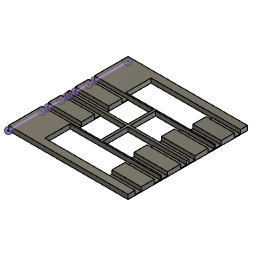
TGI_Display_Peltier_Bracket_ (Autodesk Fusion 360 design; units mm, degrees)
Autodesk Fusion 360 part; units mm, degrees
sketch "スケッチ1" plane through (0, 0, 0) normal (0, 1, 0) x (1, 0, 0)
  line L0 (-50, 50) -> (50, 50)
  line L1 (50, 50) -> (50, -50)
  line L2 (50, -50) -> (-50, -50)
  line L3 (-50, -50) -> (-50, 50)
  constraint horizontal L0
  constraint vertical L1
  constraint horizontal L2
  constraint vertical L3
extrude "押し出し1" add sketch "スケッチ1" along normal blind 3.7
sketch "スケッチ2" plane through (0, 3.7, 0) normal (0, 1, 0) x (-1, 0, 0)
  line L0 (50, 50) -> (-50, 50)
  line L1 (-50, 50) -> (-50, -50)
  line L2 (-50, -50) -> (50, -50)
  line L3 (50, -50) -> (50, 50)
  line L4 (24.7329, -44) -> (-26.2671, -44)
  line L5 (-26.2671, -44) -> (-26.2671, -23)
  line L6 (-26.2671, -23) -> (24.7329, -23)
  line L7 (24.7329, -23) -> (24.7329, -44)
  dimension "d3" = 51
  dimension "d4" = 21
  dimension "d5" = 6
  dimension "d6" = 23.7329
  constraint horizontal L4
  constraint vertical L5
  constraint horizontal L6
  constraint vertical L7
  measures "d3" distance of L4.start L4.end
  measures "d4" distance of L4.start L6.end
  measures "d5" distance of L2 L4
  measures "d6" distance of L1 L5
extrude "押し出し2" cut sketch "スケッチ2" against normal blind 3.7 contours L4 L5 L6 L7
sketch "スケッチ3" plane through (0, 3.7, 0) normal (0, 1, 0) x (-1, 0, 0)
  line L0 (-26.2671, -44) -> (-26.2671, -23)
  line L1 (-26.2671, -23) -> (24.7329, -23)
  line L2 (24.7329, -23) -> (24.7329, -44)
  line L3 (24.7329, -44) -> (-26.2671, -44)
  line L4 (50, 50) -> (-50, 50)
  line L5 (-50, 50) -> (-50, -50)
  line L6 (-50, -50) -> (50, -50)
  line L7 (50, -50) -> (50, 50)
  line L8 (-26.2671, -44) -> (-50.7671, -44)
  line L9 (-50.7671, -44) -> (-50.7671, -39)
  line L10 (-50.7671, -39) -> (-26.2671, -39)
  line L11 (-26.2671, -39) -> (-26.2671, -44)
  line L12 (-26.2671, -23) -> (-50.7671, -23)
  line L13 (-50.7671, -23) -> (-50.7671, -28)
  line L14 (-50.7671, -28) -> (-26.2671, -28)
  line L15 (-26.2671, -28) -> (-26.2671, -23)
  dimension "d9" = 24.5
  dimension "d10" = 5
  dimension "d11" = 24.5
  dimension "d12" = 5
  constraint horizontal L8
  constraint vertical L9
  constraint horizontal L10
  constraint vertical L11
  constraint coincident L0.start L3.end
  constraint horizontal L12
  constraint vertical L13
  constraint horizontal L14
  constraint vertical L15
  constraint coincident L0.end L1.start
  measures "d9" distance of L0.start L8.end
  measures "d10" distance of L0.start L10.end
  measures "d11" distance of L0.end L12.end
  measures "d12" distance of L0.end L14.end
extrude "押し出し3" cut sketch "スケッチ3" against normal blind 2.6 contours L0 L5 L8 L10 L11 | L0 L5 L12 L14 L15
sketch "スケッチ4" plane through (0, 3.7, 0) normal (0, 1, 0) x (-1, 0, 0)
  line L0 (-50, -23) -> (24.7329, -23)
  line L1 (24.7329, -23) -> (24.7329, -44)
  line L2 (24.7329, -44) -> (-50, -44)
  line L3 (-50, -44) -> (-50, -50)
  line L4 (-50, -50) -> (50, -50)
  line L5 (50, -50) -> (50, 50)
  line L6 (50, 50) -> (-50, 50)
  line L7 (-50, 50) -> (-50, -23)
  line L8 (-1, -22) -> (-22, -22)
  line L9 (-22, -22) -> (-22, -1)
  line L10 (-22, -1) -> (-1, -1)
  line L11 (-1, -1) -> (-1, -22)
  dimension "d15" = 21
  dimension "d16" = 21
  dimension "d17" = 1
  dimension "d18" = 28
  constraint horizontal L8
  constraint vertical L9
  constraint horizontal L10
  constraint vertical L11
  measures "d15" distance of L8.start L8.end
  measures "d16" distance of L8.start L10.end
  measures "d17" distance of L0 L8
  measures "d18" distance of L7 L9
extrude "押し出し4" cut sketch "スケッチ4" against normal blind 3.7 contours L8 L9 L10 L11
sketch "スケッチ5" plane through (0, 3.7, 0) normal (0, 1, 0) x (-1, 0, 0)
  line L0 (-22, -22) -> (-22, -1)
  line L1 (-22, -1) -> (-1, -1)
  line L2 (-1, -1) -> (-1, -22)
  line L3 (-1, -22) -> (-22, -22)
  line L4 (-50, -23) -> (24.7329, -23)
  line L5 (24.7329, -23) -> (24.7329, -44)
  line L6 (24.7329, -44) -> (-50, -44)
  line L7 (-50, -44) -> (-50, -50)
  line L8 (-50, -50) -> (50, -50)
  line L9 (50, -50) -> (50, 50)
  line L10 (50, 50) -> (-50, 50)
  line L11 (-50, 50) -> (-50, -23)
  line L12 (-22, -22) -> (-50, -22)
  line L13 (-50, -22) -> (-50, -17)
  line L14 (-50, -17) -> (-22, -17)
  line L15 (-22, -17) -> (-22, -22)
  line L16 (-22, -1) -> (-50, -1)
  line L17 (-50, -1) -> (-50, -6)
  line L18 (-50, -6) -> (-22, -6)
  line L19 (-22, -6) -> (-22, -1)
  dimension "d21" = 28
  dimension "d22" = 5
  dimension "d23" = 28
  dimension "d24" = 5
  constraint horizontal L12
  constraint vertical L13
  constraint horizontal L14
  constraint vertical L15
  constraint coincident L0.start L3.end
  constraint horizontal L16
  constraint vertical L17
  constraint horizontal L18
  constraint vertical L19
  constraint coincident L0.end L1.start
  measures "d21" distance of L0.start L12.end
  measures "d22" distance of L0.start L14.end
  measures "d23" distance of L0.end L16.end
  measures "d24" distance of L0.end L18.end
extrude "押し出し5" cut sketch "スケッチ5" against normal blind 2.7 contours L0 L11 L12 L13 L14 L15 | L0 L11 L16 L17 L18 L19
sketch "スケッチ6" plane through (0, 3.7, 0) normal (0, 1, 0) x (-1, 0, 0)
  line L0 (-50, -1) -> (-1, -1)
  line L1 (-1, -1) -> (-1, -22)
  line L2 (-1, -22) -> (-50, -22)
  line L3 (-50, -22) -> (-50, -23)
  line L4 (-50, -23) -> (24.7329, -23)
  line L5 (24.7329, -23) -> (24.7329, -44)
  line L6 (24.7329, -44) -> (-50, -44)
  line L7 (-50, -44) -> (-50, -50)
  line L8 (-50, -50) -> (50, -50)
  line L9 (50, -50) -> (50, 50)
  line L10 (50, 50) -> (-50, 50)
  line L11 (-50, 50) -> (-50, -1)
  line L12 (22, -22) -> (1, -22)
  line L13 (1, -22) -> (1, -1)
  line L14 (1, -1) -> (22, -1)
  line L15 (22, -1) -> (22, -22)
  dimension "d27" = 21
  dimension "d28" = 21
  dimension "d29" = 1
  dimension "d30" = 28
  constraint horizontal L12
  constraint vertical L13
  constraint horizontal L14
  constraint vertical L15
  measures "d27" distance of L12.start L12.end
  measures "d28" distance of L12.start L14.end
  measures "d29" distance of L4 L12
  measures "d30" distance of L9 L15
extrude "押し出し6" cut sketch "スケッチ6" against normal blind 3.7 contours L12 L13 L14 L15
sketch "スケッチ7" plane through (0, 3.7, 0) normal (0, 1, 0) x (-1, 0, 0)
  line L0 (1, -22) -> (1, -1)
  line L1 (1, -1) -> (22, -1)
  line L2 (22, -1) -> (22, -22)
  line L3 (22, -22) -> (1, -22)
  line L4 (-50, -1) -> (-1, -1)
  line L5 (-1, -1) -> (-1, -22)
  line L6 (-1, -22) -> (-50, -22)
  line L7 (-50, -22) -> (-50, -23)
  line L8 (-50, -23) -> (24.7329, -23)
  line L9 (24.7329, -23) -> (24.7329, -44)
  line L10 (24.7329, -44) -> (-50, -44)
  line L11 (-50, -44) -> (-50, -50)
  line L12 (-50, -50) -> (50, -50)
  line L13 (50, -50) -> (50, 50)
  line L14 (50, 50) -> (-50, 50)
  line L15 (-50, 50) -> (-50, -1)
  line L16 (22, -22) -> (50, -22)
  line L17 (50, -22) -> (50, -17)
  line L18 (50, -17) -> (22, -17)
  line L19 (22, -17) -> (22, -22)
  line L20 (22, -1) -> (50, -1)
  line L21 (50, -1) -> (50, -6)
  line L22 (50, -6) -> (22, -6)
  line L23 (22, -6) -> (22, -1)
  dimension "d33" = 28
  dimension "d34" = 5
  dimension "d35" = 28
  dimension "d36" = 5
  constraint horizontal L16
  constraint vertical L17
  constraint horizontal L18
  constraint vertical L19
  constraint coincident L2.end L3.start
  constraint horizontal L20
  constraint vertical L21
  constraint horizontal L22
  constraint vertical L23
  constraint coincident L1.end L2.start
  measures "d33" distance of L2.end L16.end
  measures "d34" distance of L2.end L18.end
  measures "d35" distance of L1.end L20.end
  measures "d36" distance of L1.end L22.end
extrude "押し出し7" cut sketch "スケッチ7" against normal blind 2.7 contours L2 L13 L16 L17 L18 L19 | L2 L13 L20 L21 L22 L23
sketch "スケッチ8" plane through (0, 3.7, 0) normal (0, 1, 0) x (-1, 0, 0)
  line L0 (1, -1) -> (50, -1)
  line L1 (50, -1) -> (50, 50)
  line L2 (50, 50) -> (-50, 50)
  line L3 (-50, 50) -> (-50, -1)
  line L4 (-50, -1) -> (-1, -1)
  line L5 (-1, -1) -> (-1, -22)
  line L6 (-1, -22) -> (-50, -22)
  line L7 (-50, -22) -> (-50, -23)
  line L8 (-50, -23) -> (24.7329, -23)
  line L9 (24.7329, -23) -> (24.7329, -44)
  line L10 (24.7329, -44) -> (-50, -44)
  line L11 (-50, -44) -> (-50, -50)
  line L12 (-50, -50) -> (50, -50)
  line L13 (50, -50) -> (50, -22)
  line L14 (50, -22) -> (1, -22)
  line L15 (1, -22) -> (1, -1)
  line L16 (-1, 1) -> (-22, 1)
  line L17 (-22, 1) -> (-22, 22)
  line L18 (-22, 22) -> (-1, 22)
  line L19 (-1, 22) -> (-1, 1)
  dimension "d39" = 21
  dimension "d40" = 21
  dimension "d41" = 2
  dimension "d42" = 28
  constraint horizontal L16
  constraint vertical L17
  constraint horizontal L18
  constraint vertical L19
  measures "d39" distance of L16.start L16.end
  measures "d40" distance of L16.start L18.end
  measures "d41" distance of L4 L16
  measures "d42" distance of L3 L17
extrude "押し出し8" cut sketch "スケッチ8" against normal blind 3.7 contours L16 L17 L18 L19
sketch "スケッチ9" plane through (0, 3.7, 0) normal (0, 1, 0) x (-1, 0, 0)
  line L0 (-22, 1) -> (-22, 22)
  line L1 (-22, 22) -> (-1, 22)
  line L2 (-1, 22) -> (-1, 1)
  line L3 (-1, 1) -> (-22, 1)
  line L4 (1, -1) -> (50, -1)
  line L5 (50, -1) -> (50, 50)
  line L6 (50, 50) -> (-50, 50)
  line L7 (-50, 50) -> (-50, -1)
  line L8 (-50, -1) -> (-1, -1)
  line L9 (-1, -1) -> (-1, -22)
  line L10 (-1, -22) -> (-50, -22)
  line L11 (-50, -22) -> (-50, -23)
  line L12 (-50, -23) -> (24.7329, -23)
  line L13 (24.7329, -23) -> (24.7329, -44)
  line L14 (24.7329, -44) -> (-50, -44)
  line L15 (-50, -44) -> (-50, -50)
  line L16 (-50, -50) -> (50, -50)
  line L17 (50, -50) -> (50, -22)
  line L18 (50, -22) -> (1, -22)
  line L19 (1, -22) -> (1, -1)
  line L20 (-22, 1) -> (-50, 1)
  line L21 (-50, 1) -> (-50, 6)
  line L22 (-50, 6) -> (-22, 6)
  line L23 (-22, 6) -> (-22, 1)
  line L24 (-22, 22) -> (-50, 22)
  line L25 (-50, 22) -> (-50, 17)
  line L26 (-50, 17) -> (-22, 17)
  line L27 (-22, 17) -> (-22, 22)
  dimension "d45" = 28
  dimension "d46" = 5
  dimension "d47" = 28
  dimension "d48" = 5
  constraint horizontal L20
  constraint vertical L21
  constraint horizontal L22
  constraint vertical L23
  constraint coincident L0.start L3.end
  constraint horizontal L24
  constraint vertical L25
  constraint horizontal L26
  constraint vertical L27
  constraint coincident L0.end L1.start
  measures "d45" distance of L0.start L20.end
  measures "d46" distance of L0.start L22.end
  measures "d47" distance of L0.end L24.end
  measures "d48" distance of L0.end L26.end
extrude "押し出し9" cut sketch "スケッチ9" against normal blind 2.7 contours L0 L7 L20 L21 L22 L23 | L0 L7 L24 L25 L26 L27
sketch "スケッチ10" plane through (0, 3.7, 0) normal (0, 1, 0) x (-1, 0, 0)
  line L0 (-1, 1) -> (-50, 1)
  line L1 (-50, 1) -> (-50, -1)
  line L2 (-50, -1) -> (-1, -1)
  line L3 (-1, -1) -> (-1, -22)
  line L4 (-1, -22) -> (-50, -22)
  line L5 (-50, -22) -> (-50, -23)
  line L6 (-50, -23) -> (24.7329, -23)
  line L7 (24.7329, -23) -> (24.7329, -44)
  line L8 (24.7329, -44) -> (-50, -44)
  line L9 (-50, -44) -> (-50, -50)
  line L10 (-50, -50) -> (50, -50)
  line L11 (50, -50) -> (50, -22)
  line L12 (50, -22) -> (1, -22)
  line L13 (1, -22) -> (1, -1)
  line L14 (1, -1) -> (50, -1)
  line L15 (50, -1) -> (50, 50)
  line L16 (50, 50) -> (-50, 50)
  line L17 (-50, 50) -> (-50, 22)
  line L18 (-50, 22) -> (-1, 22)
  line L19 (-1, 22) -> (-1, 1)
  line L20 (22, 1) -> (1, 1)
  line L21 (1, 1) -> (1, 22)
  line L22 (1, 22) -> (22, 22)
  line L23 (22, 22) -> (22, 1)
  dimension "d51" = 21
  dimension "d52" = 21
  dimension "d53" = 2
  dimension "d54" = 28
  constraint horizontal L20
  constraint vertical L21
  constraint horizontal L22
  constraint vertical L23
  measures "d51" distance of L20.start L20.end
  measures "d52" distance of L20.start L22.end
  measures "d53" distance of L14 L20
  measures "d54" distance of L15 L23
extrude "押し出し10" cut sketch "スケッチ10" against normal blind 3.7 contours L20 L21 L22 L23
sketch "スケッチ11" plane through (0, 3.7, 0) normal (0, 1, 0) x (-1, 0, 0)
  line L0 (1, 1) -> (1, 22)
  line L1 (1, 22) -> (22, 22)
  line L2 (22, 22) -> (22, 1)
  line L3 (22, 1) -> (1, 1)
  line L4 (-1, 1) -> (-50, 1)
  line L5 (-50, 1) -> (-50, -1)
  line L6 (-50, -1) -> (-1, -1)
  line L7 (-1, -1) -> (-1, -22)
  line L8 (-1, -22) -> (-50, -22)
  line L9 (-50, -22) -> (-50, -23)
  line L10 (-50, -23) -> (24.7329, -23)
  line L11 (24.7329, -23) -> (24.7329, -44)
  line L12 (24.7329, -44) -> (-50, -44)
  line L13 (-50, -44) -> (-50, -50)
  line L14 (-50, -50) -> (50, -50)
  line L15 (50, -50) -> (50, -22)
  line L16 (50, -22) -> (1, -22)
  line L17 (1, -22) -> (1, -1)
  line L18 (1, -1) -> (50, -1)
  line L19 (50, -1) -> (50, 50)
  line L20 (50, 50) -> (-50, 50)
  line L21 (-50, 50) -> (-50, 22)
  line L22 (-50, 22) -> (-1, 22)
  line L23 (-1, 22) -> (-1, 1)
  line L24 (22, 1) -> (50, 1)
  line L25 (50, 1) -> (50, 6)
  line L26 (50, 6) -> (22, 6)
  line L27 (22, 6) -> (22, 1)
  line L28 (22, 22) -> (50, 22)
  line L29 (50, 22) -> (50, 17)
  line L30 (50, 17) -> (22, 17)
  line L31 (22, 17) -> (22, 22)
  dimension "d57" = 28
  dimension "d58" = 5
  dimension "d59" = 28
  dimension "d60" = 5
  constraint horizontal L24
  constraint vertical L25
  constraint horizontal L26
  constraint vertical L27
  constraint coincident L2.end L3.start
  constraint horizontal L28
  constraint vertical L29
  constraint horizontal L30
  constraint vertical L31
  constraint coincident L1.end L2.start
  measures "d57" distance of L2.end L24.end
  measures "d58" distance of L2.end L26.end
  measures "d59" distance of L1.end L28.end
  measures "d60" distance of L1.end L30.end
extrude "押し出し11" cut sketch "スケッチ11" against normal blind 2.7 contours L2 L19 L24 L25 L26 L27 | L2 L19 L28 L29 L30 L31
sketch "スケッチ12" plane through (0, 3.7, 0) normal (0, 1, 0) x (-1, 0, 0)
  line L0 (50, 1) -> (1, 1)
  line L1 (1, 1) -> (1, 22)
  line L2 (1, 22) -> (50, 22)
  line L3 (50, 22) -> (50, 50)
  line L4 (50, 50) -> (-50, 50)
  line L5 (-50, 50) -> (-50, 22)
  line L6 (-50, 22) -> (-1, 22)
  line L7 (-1, 22) -> (-1, 1)
  line L8 (-1, 1) -> (-50, 1)
  line L9 (-50, 1) -> (-50, -1)
  line L10 (-50, -1) -> (-1, -1)
  line L11 (-1, -1) -> (-1, -22)
  line L12 (-1, -22) -> (-50, -22)
  line L13 (-50, -22) -> (-50, -23)
  line L14 (-50, -23) -> (24.7329, -23)
  line L15 (24.7329, -23) -> (24.7329, -44)
  line L16 (24.7329, -44) -> (-50, -44)
  line L17 (-50, -44) -> (-50, -50)
  line L18 (-50, -50) -> (50, -50)
  line L19 (50, -50) -> (50, -22)
  line L20 (50, -22) -> (1, -22)
  line L21 (1, -22) -> (1, -1)
  line L22 (1, -1) -> (50, -1)
  line L23 (50, -1) -> (50, 1)
  line L24 (25.5, 23) -> (-25.5, 23)
  line L25 (-25.5, 23) -> (-25.5, 44)
  line L26 (-25.5, 44) -> (25.5, 44)
  line L27 (25.5, 44) -> (25.5, 23)
  dimension "d63" = 51
  dimension "d64" = 21
  dimension "d65" = 24.5
  dimension "d66" = 1
  constraint horizontal L24
  constraint vertical L25
  constraint horizontal L26
  constraint vertical L27
  measures "d63" distance of L24.start L24.end
  measures "d64" distance of L24.start L26.end
  measures "d65" distance of L5 L25
  measures "d66" distance of L6 L24
extrude "押し出し12" cut sketch "スケッチ12" against normal blind 3.7 contours L24 L25 L26 L27
sketch "スケッチ13" plane through (0, 3.7, 0) normal (0, 1, 0) x (-1, 0, 0)
  line L0 (-25.5, 23) -> (-25.5, 44)
  line L1 (-25.5, 44) -> (25.5, 44)
  line L2 (25.5, 44) -> (25.5, 23)
  line L3 (25.5, 23) -> (-25.5, 23)
  line L4 (50, 1) -> (1, 1)
  line L5 (1, 1) -> (1, 22)
  line L6 (1, 22) -> (50, 22)
  line L7 (50, 22) -> (50, 50)
  line L8 (50, 50) -> (-50, 50)
  line L9 (-50, 50) -> (-50, 22)
  line L10 (-50, 22) -> (-1, 22)
  line L11 (-1, 22) -> (-1, 1)
  line L12 (-1, 1) -> (-50, 1)
  line L13 (-50, 1) -> (-50, -1)
  line L14 (-50, -1) -> (-1, -1)
  line L15 (-1, -1) -> (-1, -22)
  line L16 (-1, -22) -> (-50, -22)
  line L17 (-50, -22) -> (-50, -23)
  line L18 (-50, -23) -> (24.7329, -23)
  line L19 (24.7329, -23) -> (24.7329, -44)
  line L20 (24.7329, -44) -> (-50, -44)
  line L21 (-50, -44) -> (-50, -50)
  line L22 (-50, -50) -> (50, -50)
  line L23 (50, -50) -> (50, -22)
  line L24 (50, -22) -> (1, -22)
  line L25 (1, -22) -> (1, -1)
  line L26 (1, -1) -> (50, -1)
  line L27 (50, -1) -> (50, 1)
  line L28 (-25.5, 23) -> (-53.5, 23)
  line L29 (-53.5, 23) -> (-53.5, 28)
  line L30 (-53.5, 28) -> (-25.5, 28)
  line L31 (-25.5, 28) -> (-25.5, 23)
  line L32 (-25.5, 44) -> (-53.5, 44)
  line L33 (-53.5, 44) -> (-53.5, 39)
  line L34 (-53.5, 39) -> (-25.5, 39)
  line L35 (-25.5, 39) -> (-25.5, 44)
  dimension "d69" = 28
  dimension "d70" = 5
  dimension "d71" = 28
  dimension "d72" = 5
  constraint horizontal L28
  constraint vertical L29
  constraint horizontal L30
  constraint vertical L31
  constraint coincident L0.start L3.end
  constraint horizontal L32
  constraint vertical L33
  constraint horizontal L34
  constraint vertical L35
  constraint coincident L0.end L1.start
  measures "d69" distance of L0.start L28.end
  measures "d70" distance of L0.start L30.end
  measures "d71" distance of L0.end L32.end
  measures "d72" distance of L0.end L34.end
extrude "押し出し13" cut sketch "スケッチ13" against normal blind 2.7 contours L0 L9 L28 L30 L31 | L0 L9 L32 L34 L35
sketch "スケッチ14" plane through (0, 0, 0) normal (0, 1, 0) x (1, 0, 0)
extrude "押し出し14" add 2 faces at (33.6667, 1, 40.6667) (33.6667, 1, 24.6667) along direction (0, 1, 0) blind 2
extrude "押し出し15" cut 2 faces at (33.6667, 3, 40.6667) (33.6667, 3, 24.6667) along direction (0, -1, 0) blind 1.8
extrude "押し出し16" add 8 faces at (40.6667, 1, 20.3333) (40.6667, 1, 4.3333) (40.6667, 1, -2.6667) (40.6667, 1, -18.6667) (-31.3333, 1, -18.6667) (-31.3333, 1, -2.6667) (-31.3333, 1, 4.3333) (-31.3333, 1, 20.3333) along direction (0, 1, 0) blind 0.2
extrude "押し出し17" add 1 faces at (-41.5776, 3.7, -38.6667) along direction (0, 1, 0) blind 1
extrude "押し出し18" add 6 faces at (-40.6667, 3.7, -13.3333) (-40.6667, 3.7, 13.3333) (41.8333, 3.7, 35.3333) (31.3333, 3.7, 9.6667) (40.6667, 3.7, -9.6667) (42.089, 3.7, -35.3333) along direction (0, 1, 0) blind 1
sketch "スケッチ15" plane through (0, 0, 0) normal (0, 1, 0) x (1, 0, 0)
  line L0 (-50, -1) -> (-50, 1)
  line L1 (-50, 1) -> (-50, 6)
  line L2 (-50, 6) -> (-50, 17)
  line L3 (-50, 17) -> (-50, 22)
  line L4 (-50, 22) -> (-50, 50)
  line L5 (-50, 50) -> (-50, -50)
  line L6 (-50, -50) -> (-50, -22)
  line L7 (-50, -22) -> (-50, -17)
  line L8 (-50, -17) -> (-50, -6)
  line L9 (-50, -6) -> (-50, -1)
extrude "押し出し19" cut 10 faces at (33.6667, 1.2, 40.6667) (33.6667, 1.2, 24.6667) (40.6667, 1.2, 20.3333) (40.6667, 1.2, 4.3333) (40.6667, 1.2, -2.6667) (40.6667, 1.2, -18.6667) (-31.3333, 1.2, -18.6667) (-31.3333, 1.2, -2.6667) (-31.3333, 1.2, 4.3333) (-31.3333, 1.2, 20.3333) along direction (0, -1, 0) blind 0.6
extrude "押し出し20" cut 7 faces at (-41.5776, 4.7, -38.6667) (-40.6667, 4.7, 13.3333) (-40.6667, 4.7, -13.3333) (42.089, 4.7, -35.3333) (40.6667, 4.7, -9.6667) (31.3333, 4.7, 9.6667) (41.8333, 4.7, 35.3333) along direction (0, -1, 0) blind 1
extrude "押し出し21" cut 2 faces at (34.1781, 1.1, -26.3333) (34.1781, 1.1, -42.3333) along direction (0, -1, 0) blind 0.6
extrude "押し出し22" add 2 faces at (34.1781, 0.5, -42.3333) (34.1781, 0.5, -26.3333) along direction (0, 1, 0) blind 0.2
extrude "押し出し23" cut 2 faces at (34.1781, 0.7, -26.3333) (34.1781, 0.7, -42.3333) along direction (0, -1, 0) blind 0.1
